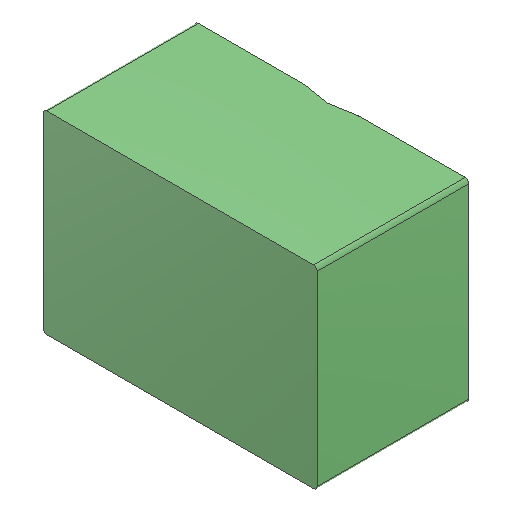
# Autodesk Inventor part: box_kit
Saved by Autodesk Inventor 2026.1 (Build 301233020, 233B)
## iProperties
Created: 2026-02-19
Part Number: box_kit
Material: LCP Plastic
Document SubType Name: Modeling
Designer: samuel
Density: 1.626 g/cm^3
Appearance: Smooth - White
Author: samuel
Autodesk Inventor part; units mm, degrees
ref_plane "YZ Plane" through (0, 0, 0) normal (1, 0, 0) x (0, 1, 0)
ref_plane "XZ Plane" through (0, 0, 0) normal (0, 1, 0) x (-1, 0, 0)
ref_plane "XY Plane" through (0, 0, 0) normal (0, 0, 1) x (1, 0, 0)
sketch "Sketch1" plane through (0, 0, 0) normal (0, 0, 1) x (1, 0, 0)
  line L0 (-51.5843, -39.0663) -> (88.4157, -39.0663)
  line L1 (88.4157, -39.0663) -> (88.4157, -9.0663)
  line L2 (88.4157, -9.0663) -> (-51.5843, -9.0663)
  line L3 (-51.5843, -9.0663) -> (-51.5843, -39.0663)
  line L4 (-53.5843, -41.0663) -> (90.4157, -41.0663)
  line L5 (90.4157, -41.0663) -> (90.4157, -7.0663)
  line L6 (90.4157, -7.0663) -> (-53.5843, -7.0663)
  line L7 (-53.5843, -7.0663) -> (-53.5843, -41.0663)
  line L8 (10.4157, -7.0663) -> (88.4157, -7.0663)
  line L9 (88.4157, -7.0663) -> (88.4157, 56.9337)
  line L10 (88.4157, 56.9337) -> (10.4157, 56.9337)
  line L11 (10.4157, 56.9337) -> (10.4157, -7.0663)
  line L12 (90.4157, 58.9337) -> (90.4157, -9.0663)
  line L13 (90.4157, -9.0663) -> (8.4157, -9.0663)
  line L14 (8.4157, -9.0663) -> (8.4157, 58.9337)
  line L15 (8.4157, 58.9337) -> (90.4157, 58.9337)
  line L16 (-53.5843, -7.0663) -> (8.4157, -7.0663)
  line L17 (8.4157, -7.0663) -> (8.4157, 58.9337)
  line L18 (8.4157, 58.9337) -> (-53.5843, 58.9337)
  line L19 (-53.5843, 58.9337) -> (-53.5843, -7.0663)
  line L20 (-51.5843, -6.0663) -> (-51.5843, 56.9337)
  line L21 (-51.5843, 56.9337) -> (9.4157, 56.9337)
  line L22 (-56.5843, -44.0663) -> (93.4157, -44.0663)
  line L23 (93.4157, -44.0663) -> (93.4157, 61.9337)
  line L24 (93.4157, 61.9337) -> (-56.5843, 61.9337)
  line L25 (-56.5843, 61.9337) -> (-56.5843, -44.0663)
  line L26 (-51.5843, -6.0663) -> (-51.5843, -9.0663)
  point P0 (0, 0)
  point P1 (90.4157, -7.0663)
  point P2 (88.4157, -7.0663)
  point P3 (10.4157, -7.0663)
  point P4 (8.4157, -7.0663)
  point P5 (-47.5843, -6.0663)
  point P6 (8.4157, 56.9337)
  point P7 (90.4157, -7.0663)
  point P8 (-51.5843, -7.0663)
  dimension "d0" = 140
  dimension "d1" = 30
  dimension "d2" = 2
  dimension "d3" = 78
  dimension "d4" = 64
  dimension "d5" = 2
  dimension "d7" = 0
  dimension "d8" = 0
  dimension "d9" = 2
  dimension "d10" = 3
  dimension "d11" = 3
  dimension "d12" = 3
  dimension "d13" = 3
  constraints: 54 end point, 12 parallel, 6 perpendicular, 4 horizontal, 7 other
  measures "d0" distance of L2.end L1.end
  measures "d1" distance of L1.end L0.end
  measures "d2" distance between parallel lines of L3 L7
  measures "d3" distance of L10.end L9.end
  measures "d4" distance of L9.end L8.end
  measures "d5" distance between parallel lines of L9 L12
  measures "d7" distance between parallel lines of L5 L12
  measures "d8" distance between parallel lines of L2 L13
  measures "d9" distance between parallel lines of L19 L20
  measures "d10" distance between parallel lines of L22 L4
  measures "d11" distance between parallel lines of L7 L25
  measures "d12" distance between parallel lines of L18 L24
  measures "d13" distance between parallel lines of L12 L23
extrude "Extrusion1" add sketch "Sketch1" along normal blind 3 contours L3 L2 L1 L0 | L0 L1 L13 L5 L4 L7 L6 L26 L3 | L26 L6 L14 L2 | L2 L14 L6 L5 L13 | L26 L20 L21 L14 L6 | L6 L19 L18 L14 L21 L20 L26 | L14 L15 L12 L6 L9 L10 L11 | L11 L10 L9 L6 | L25 L24 L23 L22
extrude "Extrusion2" add sketch "Sketch1" against normal blind 80
extrude "Extrusion3" add sketch "Sketch1" against normal blind 50 contours L0 L1 L13 L5 L4 L7 L6 L26 L3 | L26 L6 L14 L2 | L2 L14 L6 L5 L13 | L6 L19 L18 L14 L21 L20 L26 | L14 L15 L12 L6 L9 L10 L11
extrude "Extrusion4" add sketch "Sketch1" against normal blind 1 contours L3 L2 L1 L0 | L0 L1 L13 L5 L4 L7 L6 L26 L3 | L26 L6 L14 L2 | L2 L14 L6 L5 L13 | L26 L20 L21 L14 L6 | L6 L19 L18 L14 L21 L20 L26 | L14 L15 L12 L6 L9 L10 L11 | L11 L10 L9 L6
fillet "Fillet1" radius 2 4 edges at (93.4157, -44.0663, -38.5) (-56.5843, -44.0663, -38.5) (-56.5843, 61.9337, -38.5) (93.4157, 61.9337, -38.5)
sketch "Sketch3" plane through (-54.5843, 61.9337, -80) normal (0, 1, 0) x (1, 0, 0)
  line L0 (-2, 0) -> (0, 0) projected
  line L1 (-2, 0) -> (73, 0)
  line L2 (145, 0) -> (1, 0) projected
  circle A0 centre (73, 0) radius 2.5
  line L3 (73, 0) -> (73, -2.5)
  line L4 (73, -2.5) -> (87.7902, 0)
  line L5 (73, -2.5) -> (58.2098, 0)
  point P0 (54.5843, -80)
  point P1 (72.1783, -2.3611)
  point P2 (73.8217, -2.3611)
  point P3 (75.5, 0)
  point P4 (70.5, 0)
  dimension "d26" = 5
  dimension "d25" = 75
  dimension "d27" = 15
  dimension "d28" = 15
  constraints: 8 end point, 2 point on line, 1 coincident, 1 midpoint, 1 vertical, 3 other
  measures "d25" distance of L0.start L1.end
  measures "d27" distance of L3.end L4.end
  measures "d28" distance of L3.end L5.end
extrude "Extrusion6" cut sketch "Sketch3" against normal through all
fillet "Fillet2" radius 10 2 edges at (17.5941, 60.4337, -77.6389) (19.2374, 60.4337, -77.6389)
body "Solid1"
